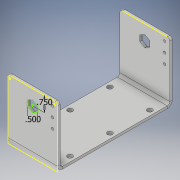
# Autodesk Inventor part: 334_18_0608_arm connection
Saved by Autodesk Inventor 2017 (Build 210142000, 142)
## iProperties
Created: 2018-01-31
Part Number: 334_18_0608_arm connection
Material: Generic
Document SubType Name: Sheet Metal
Designer: Student
Density: 1 g/cm^3
Sheet Metal Rule: Default
Appearance: Default
Author: Student
Autodesk Inventor part; units mm, degrees
ref_plane "YZ Plane" through (0, 0, 0) normal (1, 0, 0) x (0, 1, 0)
ref_plane "XZ Plane" through (0, 0, 0) normal (0, 1, 0) x (-1, 0, 0)
ref_plane "XY Plane" through (0, 0, 0) normal (0, 0, 1) x (1, 0, 0)
sketch "Sketch1" plane through (0, 0, 0) normal (0, 0, 1) x (1, 0, 0)
  line L0 (31.75, -38.1) -> (-31.75, -38.1)
  line L1 (-31.75, -38.1) -> (-31.75, 34.925)
  line L2 (-28.575, 38.1) -> (28.575, 38.1)
  line L3 (31.75, 34.925) -> (31.75, -38.1)
  line L4 (31.75, -38.1) -> (-31.75, 38.1) construction
  line L5 (-31.75, -38.1) -> (31.75, 38.1) construction
  arc A0 (31.75, 34.925) -> (28.575, 38.1) centre (28.575, 34.925) ccw
  arc A1 (-28.575, 38.1) -> (-31.75, 34.925) centre (-28.575, 34.925) ccw
  point P0 (0, 0)
  dimension "d0" = 63.5
  dimension "d1" = 76.2
  dimension "d18" = 3.175
  measures "d0" distance of L4.end L5.end
  measures "d1" distance of L0.end L4.end
  measures "d18" radius of A0
extrude "Plate1" add sketch "Sketch1" along normal blind 3.175
sketch "Sketch2" plane through (31.75, -34.925, 0) normal (0, -1, 0) x (1, 0, 0)
  line L0 (-63.5, 0) -> (0, 0)
  line L1 (0, 0) -> (0, 146.05)
  line L2 (0, 146.05) -> (-63.5, 146.05)
  line L3 (-63.5, 146.05) -> (-63.5, 0)
  constraints: 6 end point, 1 horizontal, 1 perpendicular, 1 vertical
edge flange "Flange1" height 146.05 angle 90 thickness 3.175 bend radius 3.175 thickness toward (0, -1, 0) relief tear relief width 3.175 relief depth 1.5875 edges at (0, -38.1, 3.175) wall of the first edge with corners at (-31.75, -34.925, 0) (31.75, -34.925, 0) (31.75, -34.925, 146.05) (-31.75, -34.925, 146.05)
bend "Bend1"
corner "Corner1"
sketch "Sketch3" plane through (-31.75, -34.925, 146.05) normal (0, 1, 0) x (1, 0, 0)
  circle A0 centre (6.35, 22.225) radius 3.175
  line L0 (0, 0) -> (63.5, 0) projected
  line L1 (0, 0) -> (0, 139.7) projected
  line L2 (0, 0) -> (63.5, 0) projected
  circle A1 centre (6.35, 73.025) radius 3.175
  circle A2 centre (6.35, 123.825) radius 3.175
  circle A3 centre (57.15, 22.225) radius 3.175
  circle A4 centre (57.15, 73.025) radius 3.175
  circle A5 centre (57.15, 123.825) radius 3.175
  point P0 (31.75, 146.05)
  dimension "d13" = 6.35
  dimension "d15" = 6.35
  dimension "d39" = 50.8
  dimension "d42" = 50.8
  dimension "d46" = 22.225
  constraints: 6 centre point, 1 horizontal, 1 vertical, 10 other
  measures "d13" diameter of A0
  measures "d15" distance from line of L1 A0.centre
  measures "d39" distance of A0.centre A1.centre
  measures "d42" distance of A0.centre A3.centre
  measures "d46" distance from line of L0 A0.centre
extrude "Cut1" cut sketch "Sketch3" against normal blind 3.175
sketch "Sketch4" plane through (0, 0, 3.175) normal (0, 0, 1) x (1, 0, 0)
  line L0 (-28.575, 38.1) -> (28.575, 38.1) projected
sketch "Sketch5" plane through (-31.75, -38.1, 146.05) normal (0, 0, 1) x (1, 0, 0)
  line L0 (0, 6.35) -> (0, 73.025) projected
  arc A0 (3.175, 76.2) -> (0, 73.025) centre (3.175, 73.025) ccw projected
  line L1 (3.175, 76.2) -> (60.325, 76.2) projected
  arc A1 (63.5, 73.025) -> (60.325, 76.2) centre (60.325, 73.025) ccw projected
  line L2 (63.5, 73.025) -> (63.5, 6.35) projected
  line L3 (0, 0) -> (63.5, 0) projected
  line L4 (0, 3.175) -> (0, 0) projected
  line L5 (63.5, 3.175) -> (63.5, 0) projected
  line L6 (63.5, 3.175) -> (63.5, 6.35) projected
  line L7 (0, 3.175) -> (0, 6.35) projected
  line L8 (31.75, 64.4823) -> (38.1, 60.8162)
  line L9 (38.1, 60.8162) -> (38.1, 53.4838)
  line L10 (38.1, 53.4838) -> (31.75, 49.8177)
  line L11 (31.75, 49.8177) -> (25.4, 53.4838)
  line L12 (25.4, 53.4838) -> (25.4, 60.8162)
  line L13 (25.4, 60.8162) -> (31.75, 64.4823)
  point P0 (31.75, 57.15)
  dimension "d51" = 12.7
  dimension "d52" = 19.05
  constraints: 12 end point, 13 other
  measures "d51" distance between parallel lines of L9 L12
  measures "d52" distance from line of L1 point (31.75, 57.15)
sketch "Sketch6" plane through (31.75, -38.1, 142.875) normal (0, 0, 1) x (1, 0, 0)
  line L0 (-63.5, 0) -> (0, 0)
  line L1 (0, 0) -> (0, 76.2)
  line L2 (0, 76.2) -> (-63.5, 76.2)
  line L3 (-63.5, 76.2) -> (-63.5, 0)
  constraints: 6 end point, 1 horizontal, 1 perpendicular, 1 vertical
edge flange "Flange2" height 76.2 angle 90 thickness 3.175 bend radius 3.175 thickness toward (0, 0, 1) relief tear relief width 3.175 relief depth 1.5875 edges at (0, -34.925, 146.05) wall of the first edge with corners at (-31.75, -38.1, 142.875) (31.75, -38.1, 142.875) (31.75, 38.1, 142.875) (-31.75, 38.1, 142.875)
bend "Bend2"
corner "Corner2"
fillet "Corner Round1" radius 3.175 2 edges at (-31.75, 38.1, 144.4625) (31.75, 38.1, 144.4625)
extrude "Cut5" cut sketch "Sketch5" against normal blind 3.175 contours L8 L9 L10 L11 L12 L13
sketch "Sketch7" plane through (0, 0, 0) normal (0, 0, -1) x (-1, 0, 0)
  line L0 (0, 26.3823) -> (6.35, 22.7162) projected
  line L1 (-6.35, 22.7162) -> (0, 26.3823) projected
  line L2 (-6.35, 15.3838) -> (-6.35, 22.7162) projected
  line L3 (0, 11.7177) -> (-6.35, 15.3838) projected
  line L4 (6.35, 15.3838) -> (0, 11.7177) projected
  line L5 (6.35, 22.7162) -> (6.35, 15.3838) projected
  point P0 (0, 0)
extrude "Cut6" cut sketch "Sketch7" against normal blind 3.175
sketch "Sketch8" plane through (0, 0, 0) normal (0, 0, -1) x (-1, 0, 0)
  circle A0 centre (-25.273, 31.75) radius 1.5875
  circle A1 centre (-25.273, 19.05) radius 1.5875
  circle A2 centre (-25.273, 6.35) radius 1.5875
  line L0 (31.75, -31.75) -> (31.75, 34.925) projected
  line L1 (28.575, 38.1) -> (-28.575, 38.1) projected
  line L2 (-31.75, 34.925) -> (-31.75, -31.75) projected
  point P0 (0, 0)
  dimension "d57" = 3.175
  dimension "d58" = 3.175
  dimension "d59" = 3.175
  dimension "d61" = 6.35
  dimension "d62" = 12.7
  dimension "d63" = 12.7
  dimension "d68" = 6.477
  constraints: 3 centre point, 2 vertical alignment
  measures "d57" diameter of A0
  measures "d58" diameter of A1
  measures "d59" diameter of A2
  measures "d61" distance from line of L1 A0.centre
  measures "d62" distance of A0.centre A1.centre
  measures "d63" distance of A1.centre A2.centre
  measures "d68" distance from line of L2 A0.centre
extrude "Cut7" cut sketch "Sketch8" against normal blind 3.175
sketch "Sketch9" plane through (-31.75, -31.75, 146.05) normal (0, 0, 1) x (1, 0, 0)
  circle A0 centre (57.023, 38.1) radius 1.5875 projected
  circle A1 centre (57.023, 50.8) radius 1.5875 projected
  circle A2 centre (57.023, 63.5) radius 1.5875 projected
  circle A3 centre (57.023, 63.5) radius 1.5875
  circle A4 centre (57.023, 50.8) radius 1.5875
  circle A5 centre (57.023, 38.1) radius 1.5875
  point P0 (31.75, 31.75)
  constraints: 3 centre point, 3 coincident, 3 concentric
extrude "Cut8" cut sketch "Sketch9" against normal blind 3.175
equation "\"d16\" = Thickness"
equation "\"d53\" = Thickness"
equation "\"d55\" = Thickness"
equation "\"d64\" = Thickness"
equation "\"d66\" = Thickness"
equation "\"d3\" = BendReliefWidth"
equation "\"d4\" = BendReliefDepth"
equation "\"d5\" = MinimumRemnant"
equation "\"d6\" = BendRadius"
equation "\"d9\" = BendRadius"
equation "\"d10\" = CornerReliefSize"
equation "\"d11\" = GapSize"
equation "\"d12\" = JacobiRadiusSize"
equation "\"d24\" = BendReliefWidth"
equation "\"d25\" = BendReliefDepth"
equation "\"d26\" = MinimumRemnant"
equation "\"d27\" = BendRadius"
equation "\"d30\" = BendRadius"
equation "\"d31\" = CornerReliefSize"
equation "\"d32\" = GapSize"
equation "\"d33\" = JacobiRadiusSize"
equation "\"BendRadius\" = Thickness"
equation "\"BendReliefWidth\" = Thickness"
equation "\"BendReliefDepth\" = 0.5 * Thickness"
equation "\"CornerReliefSize\" = 4 * Thickness"
equation "\"MinimumRemnant\" = 2 * Thickness"
equation "\"TransitionRadius\" = BendRadius"
equation "\"JacobiRadiusSize\" = BendRadius"
equation "\"GapSize\" = Thickness"
equation "\"d2\" = BendRadius"
equation "\"Thickness\" = 3.175"
body "Solid1"
